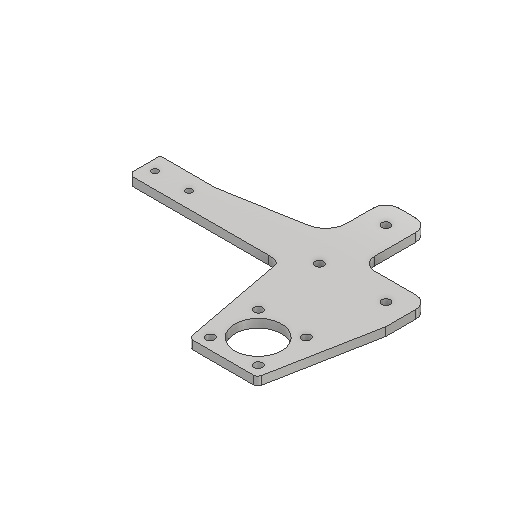
# Autodesk Inventor part: LC_ALU_4mm_Heatbed_Frame_Linear_Bearing_Mounting_Bracket_Cable_Chain
Saved by Autodesk Inventor 2026.1 (Build 301233000, 233)
## iProperties
Created: 2016-06-21
Part Number: LC_ALU_4mm_Heatbed_Frame_Linear_Bearing_Mounting_Bracket_Cable_Chain
Material: Ogólny
Document SubType Name: Modeling
Designer: Andrzej
Density: 1 g/cm^3
Appearance: Obrobione - aluminium
Mass: 18.2722 g
Surface Area: 114.031 cm^2
Volume: 18.2722 cm^3
Author: Andrzej
Autodesk Inventor part; units mm, degrees
ref_plane "YZ Plane" through (0, 0, 0) normal (1, 0, 0) x (0, 1, 0)
ref_plane "XZ Plane" through (0, 0, 0) normal (0, 1, 0) x (-1, 0, 0)
ref_plane "XY Plane" through (0, 0, 0) normal (0, 0, 1) x (1, 0, 0)
sketch "Szkic1" plane through (0, 0, 0) normal (0, 0, 1) x (1, 0, 0)
  line L0 (-25.3316, -15.5729) -> (26.0684, -15.5729)
  line L1 (26.0684, -15.5729) -> (26.0684, 35.4271)
  line L2 (26.0684, 35.4271) -> (26.0684, 35.4271)
  line L3 (26.0684, 35.4271) -> (26.0684, 55.4271)
  line L4 (26.0684, 55.4271) -> (-5.3316, 55.4271)
  line L5 (-5.3316, 55.4271) -> (-5.3316, 86.8271)
  line L6 (-5.3316, 86.8271) -> (-25.3316, 86.8271)
  line L7 (-25.3316, -15.5729) -> (-25.3316, 86.8271)
  line L8 (-15.6316, 16.9271) -> (16.3684, 16.9271)
  line L9 (16.3684, 16.9271) -> (16.3684, -15.0729)
  line L10 (16.3684, -15.0729) -> (-15.6316, -15.0729)
  line L11 (-15.6316, -15.0729) -> (-15.6316, 16.9271)
  circle A0 centre (0.3684, 0.9271) radius 11
  circle A1 centre (0.3684, 0.9271) radius 16
  line L12 (-25.3316, 51.9271) -> (-96.8316, 51.9271)
  line L13 (-96.8316, 51.9271) -> (-96.8316, 36.9271)
  line L14 (-96.8316, 36.9271) -> (-25.3316, 36.9271)
  line L15 (-25.3316, 36.9271) -> (-25.3316, 51.9271)
  point P0 (0, 0)
  point P1 (-10.9453, 12.2408)
  point P2 (11.6821, 12.2408)
  point P3 (11.6821, -10.3866)
  point P4 (-10.9453, -10.3866)
  point P5 (16.0684, 45.4271)
  point P6 (-15.3316, 76.8271)
  point P7 (-15.3316, 45.4271)
  point P8 (-91.8316, 44.4271)
  point P9 (-75.8316, 44.4271)
  dimension "d0" = 20
  dimension "d1" = 20
  dimension "d2" = 51.4
  dimension "d3" = 51.4
  dimension "d4" = 34.5
  dimension "d5" = 25.7
  dimension "d6" = 51.4
  dimension "d7" = 51
  dimension "d8" = 32
  dimension "d9" = 32
  dimension "d10" = 16
  dimension "d11" = 16
  dimension "d12" = 22
  dimension "d13" = 32
  dimension "d23" = 10
  dimension "d24" = 10
  dimension "d25" = 10
  dimension "d26" = 10
  dimension "d27" = 10
  dimension "d28" = 10
  dimension "d45" = 71.5
  dimension "d46" = 15
  dimension "d47" = 18.5
  dimension "d57" = 5
  dimension "d58" = 16
  dimension "d59" = 7.5
  dimension "d60" = 7.5
  constraints: 32 end point, 8 perpendicular, 4 parallel, 4 point on circle, 3 horizontal, 2 centre point, 2 coincident, 1 point on line, 1 vertical
  measures "d0" distance between parallel lines of L7 L5
  measures "d1" distance of L2.end L3.end
  measures "d2" distance between parallel lines of L2 L6
  measures "d3" distance between parallel lines of L7 L3
  measures "d4" distance from line of L2 point (0.368, 0.927)
  measures "d5" distance from line of L7 point (0.368, 0.927)
  measures "d6" distance between parallel lines of L1 L7
  measures "d7" distance between parallel lines of L0 L2
  measures "d8" distance of L9.end L10.end
  measures "d9" distance of L8.end L9.end
  measures "d10" distance from line of L8 point (0.368, 0.927)
  measures "d11" distance from line of L11 point (0.368, 0.927)
  measures "d12" diameter of A0
  measures "d13" diameter of A1
  measures "d23" distance from line of L6 point (-15.332, 76.827)
  measures "d24" distance from line of L3 point (16.068, 45.427)
  measures "d25" distance from line of L4 point (16.068, 45.427)
  measures "d26" distance from line of L5 point (-15.332, 76.827)
  measures "d27" distance from line of L4 point (-15.332, 45.427)
  measures "d28" distance from line of L5 point (-15.332, 45.427)
  measures "d45" distance of L14.end L13.end
  measures "d46" distance of L12.end L13.end
  measures "d47" distance between parallel lines of L4 L14
  measures "d57" distance from line of L13 point (-91.832, 44.427)
  measures "d58" distance of point (-91.832, 44.427) point (-75.832, 44.427)
  measures "d59" distance from line of L14 point (-91.832, 44.427)
  measures "d60" distance from line of L14 point (-75.832, 44.427)
extrude "Wyciągnięcie proste1" add sketch "Szkic1" along normal blind 4 contours L7 L6 L5 L4 L3 L1 L0 | L8 A1 L11 | L8 L9 A1 | A1 | A1 L10 L11 | L9 L10 A1
hole "Otwór1" at (0.3684, 0.9271, 0) at (-10.9453, 12.2408, 0) at (11.6821, 12.2408, 0) at (11.6821, -10.3866, 0) at (-10.9453, -10.3866, 0) direction (0, 0, 1) diameter 4 end through all
hole "Otwór2" at (16.0684, 45.4271, 0) at (-15.3316, 76.8271, 0) at (-15.3316, 45.4271, 0) direction (0, 0, 1) diameter 4 end through all
chamfer "Faza1" distance 51 distance2 9.7 1 edges at (-25.3316, -15.5729, 2) measured on face at (-25.3316, 18.5605, 1.3333)
chamfer "Faza2" distance 51 distance2 9.7 1 edges at (26.0684, -15.5729, 2) measured on face at (26.0684, 31.7605, 1.3333)
fillet "Zaokrąglenie1" radius 2 2 edges at (-15.6316, -15.5729, 2) (16.3684, -15.5729, 2)
fillet "Zaokrąglenie2" radius 6 4 edges at (-5.3316, 55.4271, 2) (26.0684, 55.4271, 2) (-5.3316, 86.8271, 2) (-25.3316, 86.8271, 2)
extrude "Wyciągnięcie proste2" add sketch "Szkic1" along normal blind 4 contours L14 L13 L12 L7
chamfer "Faza3" distance 8 distance2 45.5 1 edges at (-25.3316, 51.9271, 2) measured on face at (-25.3316, 61.5605, 1.3333)
fillet "Zaokrąglenie4" radius 10 2 edges at (-25.3316, 59.9271, 2) (-25.3316, 36.9271, 2)
chamfer "Faza4" distance 2 angle 45 1 edges at (-96.8316, 36.9271, 2)
hole "Otwór3" at (-91.8316, 44.4271, 0) at (-75.8316, 44.4271, 0) direction (0, 0, 1) diameter 3 end through all
equation "\"d1\" = d0"
equation "\"d2\" = d6"
equation "\"d3\" = d6"
equation "\"d6\" = 2 * d5"
equation "\"d10\" = 0.5 * d9"
equation "\"d11\" = 0.5 * d8"
equation "\"d25\" = 0.5 * d1"
equation "\"d26\" = 0.5 * d0"
equation "\"d27\" = d25"
equation "\"d28\" = d26"
